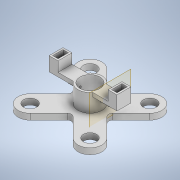
# Autodesk Inventor part: PISTON_CYLINDER
Saved by Autodesk Inventor 2021 (Build 250183000, 183)
## iProperties
Created: 2021-03-18
Part Number: PISTON_CYLINDER
Material: Generic
Document SubType Name: Modeling
Designer: Sihan
Density: 1 g/cm^3
Appearance: Default
Author: Sihan
Autodesk Inventor part; units mm, degrees
ref_plane "XZ Plane" through (0, 0, 0) normal (0, 1, 0) x (-1, 0, 0)
ref_plane "XY Plane" through (0, 0, 0) normal (0, 0, 1) x (1, 0, 0)
sketch "Sketch1" plane through (0, 0, 0) normal (0, 1, 0) x (-1, 0, 0)
  circle A0 centre (0, 0) radius 5
  circle A1 centre (0, 0) radius 6
  dimension "d0" = 10
  dimension "d1" = 12
  constraints: 2 centre point, 2 coincident
  measures "d0" diameter of A0
  measures "d1" diameter of A1
extrude "Extrusion1" add sketch "Sketch1" along normal blind 8
sketch "Sketch2" plane through (0, 0, 0) normal (0, -1, 0) x (1, 0, 0)
  circle A0 centre (0, 0) radius 6
  constraints: 1 centre point, 1 coincident
extrude "Extrusion2" add sketch "Sketch2" along normal blind 1
sketch "Sketch3" plane through (0, 0, 0) normal (1, 0, 0) x (0, 1, 0)
  line L0 (-1, -6) -> (8, -6) construction
  line L1 (3.5, -6) -> (3.5, -10.9268) construction
  line L2 (4.4, -6) -> (4.4, -8)
  line L3 (4.4, -8) -> (5, -8)
  line L4 (5, -8) -> (4.4, -9.5)
  line L5 (4.4, -9.5) -> (4.1, -9.5)
  line L6 (4.1, -9.5) -> (4.1, -6)
  point P0 (0, 0)
  dimension "d6" = 0.9
  dimension "d7" = 1.5
  dimension "d8" = 0.6
  dimension "d9" = 2
  dimension "d10" = 1.5
  dimension "d13" = 3.5
  dimension "d14" = 0.9
  constraints: 12 end point, 2 perpendicular, 2 point on line, 2 vertical, 1 horizontal, 1 midpoint
  measures "d6" distance from line of L4.end L1
  measures "d7" distance from line of L1 L3.end
  measures "d8" distance between parallel lines of L1 L6
  measures "d9" vertical distance of L6.end L3.end
  measures "d10" distance from line of L4.end L3
  measures "d13" distance from line of point (0, 0) L1
  measures "d14" distance from line of L1 L2.end
revolve "Revolution1" [suppressed]
sketch "Sketch4" plane through (0, 3.5, -9.5) normal (0, 0, -1) x (-1, 0, 0)
  circle A0 centre (0, 0) radius 0.6 projected
  circle A1 centre (0, 0) radius 0.6
  point P0 (0, -3.5)
  constraints: 1 centre point, 1 coincident
extrude "Extrusion3" [suppressed]
pattern_circular "Circular Pattern1" [suppressed]
sketch "Sketch7" plane through (0, 8, 0) normal (0, 1, 0) x (1, 0, 0)
  line L0 (-13.525, 2.5) -> (-16.025, 2.5)
  line L1 (-16.025, 2.5) -> (-16.025, -2.5)
  line L2 (-16.025, -2.5) -> (-13.525, -2.5)
  line L3 (-13.525, -2.5) -> (-13.525, 2.5)
  line L4 (13.525, 2.5) -> (16.025, 2.5)
  line L5 (16.025, 2.5) -> (16.025, -2.5)
  line L6 (16.025, -2.5) -> (13.525, -2.5)
  line L7 (13.525, -2.5) -> (13.525, 2.5)
  line L8 (-17.025, 3.5) -> (-12.525, 3.5)
  line L9 (-12.525, 3.5) -> (-12.525, -3.5)
  line L10 (-12.525, -3.5) -> (-17.025, -3.5)
  line L11 (-17.025, -3.5) -> (-17.025, 3.5)
  line L12 (17.025, 3.5) -> (12.525, 3.5)
  line L13 (12.525, 3.5) -> (12.525, -3.5)
  line L14 (12.525, -3.5) -> (17.025, -3.5)
  line L15 (17.025, -3.5) -> (17.025, 3.5)
  point P0 (0, 0)
  dimension "d30" = 2.5
  dimension "d31" = 5
  dimension "d32" = 2.5
  dimension "d33" = 5
  dimension "d34" = 2.5
  dimension "d35" = 2.5
  dimension "d38" = 1
  dimension "d39" = 1
  dimension "d44" = 25.05
  dimension "d45" = 12.525
  constraints: 32 end point, 8 parallel, 4 perpendicular, 2 horizontal, 6 other
  measures "d30" distance of L0.start L0.end
  measures "d31" distance of L2.end L0.start
  measures "d32" distance of L4.start L4.end
  measures "d33" distance of L4.end L5.end
  measures "d34" vertical distance of point (0, 0) L0.start
  measures "d35" vertical distance of point (0, 0) L4.start
  measures "d38" distance between parallel lines of L8 L0
  measures "d39" distance between parallel lines of L12 L4
  measures "d44" distance between parallel lines of L13 L9
  measures "d45" distance from line of point (0, 0) L9
sketch "Sketch8" plane through (0, 8, 0) normal (0, 1, 0) x (1, 0, 0)
  line L0 (17.025, 3.5) -> (17.025, -3.5)
  line L1 (-17.025, -3.5) -> (-17.025, 3.5)
  line L2 (-17.025, 3.5) -> (-4.8734, 3.5)
  line L3 (4.8734, 3.5) -> (17.025, 3.5)
  arc A0 (-4.8734, 3.5) -> (-4.8734, -3.5) centre (0, 0) ccw
  arc A1 (4.8734, -3.5) -> (4.8734, 3.5) centre (0, 0) ccw
  line L4 (17.025, -3.5) -> (4.8734, -3.5)
  line L5 (-4.8734, -3.5) -> (-17.025, -3.5)
  constraints: 12 end point, 5 parallel, 4 point on circle, 2 centre point, 2 horizontal, 2 perpendicular, 1 coincident
extrude "Extrusion5" add sketch "Sketch8" against normal blind 2
extrude "Extrusion6" add sketch "Sketch7" along normal blind 5
ref_plane "Work Plane1" through (10, 0, 0) normal (1, 0, 0) x (0, 1, 0)
sketch "Sketch10" plane through (10, 0, 0) normal (1, 0, 0) x (0, 1, 0)
  circle A0 centre (3.5, 0) radius 0.9
  point P0 (0, 0)
  dimension "d47" = 1.8
  dimension "d48" = 3.5
  constraints: 1 centre point
  measures "d47" diameter of A0
  measures "d48" distance of point (0, 0) A0.centre
extrude "Extrusion7" add sketch "Sketch10" against normal up to next
sketch "Sketch11" plane through (10, 3.5, 0) normal (1, 0, 0) x (0, 0, -1)
  circle A0 centre (0, 0) radius 0.6
  point P0 (0, -3.5)
  dimension "d51" = 1.2
  constraints: 1 centre point
  measures "d51" diameter of A0
extrude "Extrusion8" cut sketch "Sketch11" against normal up to next
pattern_circular "Circular Pattern2" count 2 over 360 about axis through (0, -10, 0) along (0, 1, 0) of "Extrusion8", "Extrusion7"
sketch "Sketch12" plane through (0, -1, 0) normal (0, -1, 0) x (1, 0, 0)
  circle A0 centre (-15, 15) radius 3.3
  circle A1 centre (15, 15) radius 3.3
  circle A2 centre (15, -15) radius 3.3
  circle A3 centre (-15, -15) radius 3.3
  line L0 (-15, 15) -> (15, -15) construction
  arc A4 (-10.7574, 19.2426) -> (-19.2426, 10.7574) centre (-15, 15) ccw
  arc A5 (10.7574, -19.2426) -> (19.2426, -10.7574) centre (15, -15) ccw
  line L1 (-15, -15) -> (15, 15) construction
  arc A6 (-19.2426, -10.7574) -> (-10.7574, -19.2426) centre (-15, -15) ccw
  arc A7 (19.2426, 10.7574) -> (10.7574, 19.2426) centre (15, 15) ccw
  line L2 (10.7574, 19.2426) -> (1.4142, 9.8995)
  line L3 (-9.8995, -1.4142) -> (-19.2426, -10.7574)
  line L4 (-19.2426, 10.7574) -> (-9.8995, 1.4142)
  line L5 (1.4142, -9.8995) -> (10.7574, -19.2426)
  line L6 (-10.7574, -19.2426) -> (-1.4142, -9.8995)
  line L7 (9.8995, 1.4142) -> (19.2426, 10.7574)
  line L8 (19.2426, -10.7574) -> (9.8995, -1.4142)
  line L9 (-1.4142, 9.8995) -> (-10.7574, 19.2426)
  arc A8 (-1.4142, 9.8995) -> (1.4142, 9.8995) centre (0, 11.3137) ccw
  arc A9 (-9.8995, -1.4142) -> (-9.8995, 1.4142) centre (-11.3137, 0) ccw
  arc A10 (1.4142, -9.8995) -> (-1.4142, -9.8995) centre (0, -11.3137) ccw
  arc A11 (9.8995, 1.4142) -> (9.8995, -1.4142) centre (11.3137, 0) ccw
  point P0 (0, 0)
  point P1 (0, 0)
  point P2 (0, 0)
  dimension "d57" = 15
  dimension "d58" = 15
  dimension "d59" = 15
  dimension "d60" = 15
  dimension "d61" = 15
  dimension "d62" = 15
  dimension "d63" = 15
  dimension "d64" = 15
  dimension "d65" = 6.6
  dimension "d66" = 6.6
  dimension "d67" = 6.6
  dimension "d68" = 6.6
  dimension "d69" = 6
  dimension "d70" = 6
  dimension "d71" = 2
  constraints: 24 end point, 24 tangent, 16 point on circle, 12 centre point, 8 parallel, 3 equal radius, 2 midpoint
  measures "d57" horizontal distance of point (0, 0) L0.start
  measures "d58" horizontal distance of point (0, 0) L0.start
  measures "d59" horizontal distance of point (0, 0) L1.start
  measures "d60" horizontal distance of point (0, 0) L1.start
  measures "d61" horizontal distance of point (0, 0) L0.end
  measures "d62" horizontal distance of point (0, 0) L0.end
  measures "d63" horizontal distance of point (0, 0) L1.end
  measures "d64" horizontal distance of point (0, 0) L1.end
  measures "d65" diameter of A0
  measures "d66" diameter of A1
  measures "d67" diameter of A2
  measures "d68" diameter of A3
  measures "d69" radius of A4
  measures "d70" radius of A7
  measures "d71" radius of A8
extrude "Extrusion9" add sketch "Sketch12" along normal blind 3
sketch "Sketch13" plane through (0, 13, 0) normal (0, 1, 0) x (1, 0, 0)
  line L0 (-13.525, 2.5) -> (-16.025, 2.5) projected
  line L1 (-16.025, 2.5) -> (-16.025, -2.5) projected
  line L2 (-16.025, -2.5) -> (-13.525, -2.5) projected
  line L3 (-13.525, -2.5) -> (-13.525, 2.5) projected
  line L4 (13.525, 2.5) -> (13.525, -2.5) projected
  line L5 (13.525, -2.5) -> (16.025, -2.5) projected
  line L6 (16.025, -2.5) -> (16.025, 2.5) projected
  line L7 (16.025, 2.5) -> (13.525, 2.5) projected
  line L8 (-16.125, 2.6) -> (-13.425, 2.6)
  line L9 (-13.425, 2.6) -> (-13.425, -2.6)
  line L10 (-13.425, -2.6) -> (-16.125, -2.6)
  line L11 (-16.125, -2.6) -> (-16.125, 2.6)
  line L12 (13.425, 2.6) -> (13.425, -2.6)
  line L13 (13.425, -2.6) -> (16.125, -2.6)
  line L14 (16.125, -2.6) -> (16.125, 2.6)
  line L15 (16.125, 2.6) -> (13.425, 2.6)
  point P0 (0, 0)
  dimension "d74" = 0.1
  dimension "d75" = 0.1
  constraints: 16 end point, 6 other
  measures "d74" distance between parallel lines of L0 L8
  measures "d75" distance between parallel lines of L15 L7
extrude "Extrusion10" cut sketch "Sketch13" against normal up to surface (5 mm away) contours L3 L2 L1 L0 | L7 L6 L5 L4 | L8 L9 L10 L11 | L15 L14 L13 L12
body "Solid1"
